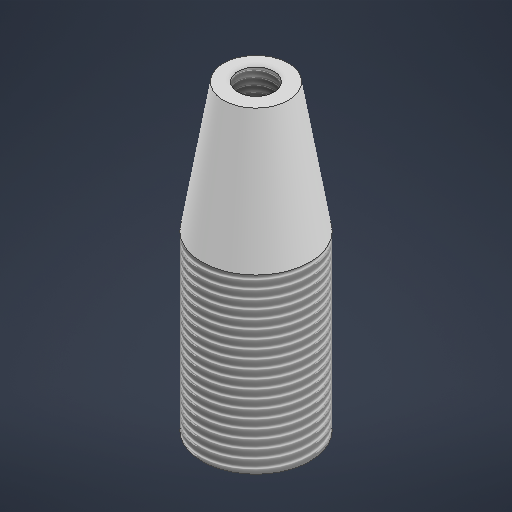
# Autodesk Inventor part: Output link probe hub
Saved by Autodesk Inventor 2026.3 (Build 303398000, 398)
## iProperties
Created: 2026-07-24
Part Number: Output link probe hub
Material: Generic
Document SubType Name: Sheet Metal
Designer: matot
Density: 1 g/cm^3
Sheet Metal Rule: Default_mm
Appearance: Default
Author: matot
Autodesk Inventor part; units mm, degrees
ref_plane "YZ Plane" through (0, 0, 0) normal (1, 0, 0) x (0, 1, 0)
ref_plane "XZ Plane" through (0, 0, 0) normal (0, 1, 0) x (-1, 0, 0)
ref_plane "XY Plane" through (0, 0, 0) normal (0, 0, 1) x (1, 0, 0)
sketch "Sketch1" plane through (0, 0, 0) normal (0, 0, 1) x (1, 0, 0)
  line L0 (0, 30) -> (0, 0)
  line L1 (0, 0) -> (12.5, 0)
  line L2 (0, 30) -> (7.5, 30)
  line L3 (7.5, 30) -> (12.5, 0)
  dimension "d0" = 7.5
  dimension "d1" = 12.5
  dimension "d2" = 30
  constraints: 8 end point, 1 horizontal, 1 vertical
  measures "d0" distance of L0.start L2.end
  measures "d1" distance of L0.end L1.end
  measures "d2" distance of L0.start L0.end
revolve "Revolution1" add sketch "Sketch1" angle 360 about axis through (0, 30, 0) along (0, -1, 0)
sketch "Sketch2" plane through (0, 0, 0) normal (0, -1, 0) x (1, 0, 0)
  circle A0 centre (0, 0) radius 12.5
  constraints: 1 centre point, 1 coincident
extrude "Extrusion1" add sketch "Sketch2" along normal blind 40
thread "Thread1" size "M25x2" class "6g" standard "ANSI Metric M Profile" full length
thread "Thread2" size "M25x2" class "6g" standard "ISO Metric profile" full length
sketch "Sketch3" plane through (0, 30, 0) normal (0, 1, 0) x (1, 0, 0)
  circle A0 centre (0, 0) radius 5
  dimension "d10" = 10
  constraints: 2 coincident, 1 centre point
  measures "d10" diameter of A0
hole "Hole1" at (0, 30, 0) direction (0, -1, 0) diameter 8.376 depth 27.3 tip angle 118 thread size "M10x1.5" class "6H" standard "ISO Metric profile"
equation "\"BendRadius\" = Thickness"
equation "\"BendReliefWidth\" = Thickness"
equation "\"BendReliefDepth\" = 0.5 * Thickness"
equation "\"CornerReliefSize\" = 4 * Thickness"
equation "\"MinimumRemnant\" = 2 * Thickness"
equation "\"TransitionRadius\" = BendRadius"
equation "\"JacobiRadiusSize\" = BendRadius"
equation "\"GapSize\" = Thickness"
equation "\"Thickness\" = 0.5"
body "Solid1"
